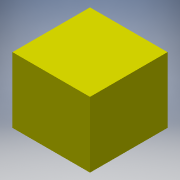
# Autodesk Inventor part: 2018 power cube
Saved by Autodesk Inventor 2018 (Build 220112000, 112)
## iProperties
Created: 2018-01-16
Part Number: 2018 power cube
Material: Generic
Document SubType Name: Modeling
Designer: Apple
Density: 1 g/cm^3
Appearance: Default
Author: Apple
Autodesk Inventor part; units mm, degrees
ref_plane "YZ Plane" through (0, 0, 0) normal (1, 0, 0) x (0, 1, 0)
ref_plane "XZ Plane" through (0, 0, 0) normal (0, 1, 0) x (-1, 0, 0)
ref_plane "XY Plane" through (0, 0, 0) normal (0, 0, 1) x (1, 0, 0)
sketch "Sketch1" plane through (0, 0, 0) normal (0, 0, 1) x (1, 0, 0)
  line L0 (-338.3031, 181.5744) -> (-8.1031, 181.5744)
  line L1 (-8.1031, 181.5744) -> (-8.1031, 460.9744)
  line L2 (-8.1031, 460.9744) -> (-338.3031, 460.9744)
  line L3 (-338.3031, 460.9744) -> (-338.3031, 181.5744)
  line L4 (-338.3031, 181.5744) -> (-8.1031, 460.9744) construction
  line L5 (-8.1031, 181.5744) -> (-338.3031, 460.9744) construction
  point P0 (0, 0)
  point P1 (-173.2031, 321.2744)
  dimension "d0" = 330.2
  dimension "d1" = 279.4
  constraints: 12 end point, 2 midpoint, 2 parallel, 1 horizontal, 1 perpendicular
  measures "d0" distance of L2.end L1.end
  measures "d1" distance of L1.end L0.end
extrude "Extrusion1" add sketch "Sketch1" along normal blind 330.2
body "Solid1"
